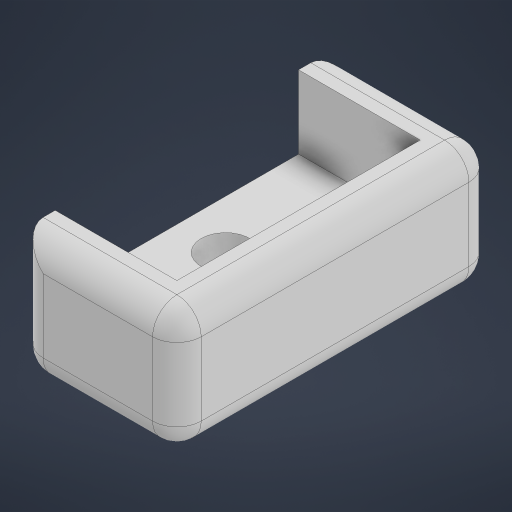
# Autodesk Inventor part: 2
Saved by Autodesk Inventor 2024 (Build 280153000, 153)
## iProperties
Created: 2023-05-05
Part Number: 2
Material: Типовые
Document SubType Name: Modeling
Designer: user
Density: 1 g/cm^3
Appearance: По умолчанию
Author: user
Autodesk Inventor part; units mm, degrees
ref_plane "YZ Plane" through (0, 0, 0) normal (1, 0, 0) x (0, 1, 0)
ref_plane "XZ Plane" through (0, 0, 0) normal (0, 1, 0) x (-1, 0, 0)
ref_plane "XY Plane" through (0, 0, 0) normal (0, 0, 1) x (1, 0, 0)
sketch "Эскиз1" plane through (0, 0, 0) normal (0, 0, 1) x (1, 0, 0)
  line L0 (0, 0) -> (10, 0)
  line L1 (10, 0) -> (10, 20)
  line L2 (10, 20) -> (0, 20)
  line L3 (0, 20) -> (0, 0)
  circle A0 centre (4, 10) radius 2
  point P0 (10, 10)
  dimension "d0" = 10
  dimension "d1" = 4
  dimension "d2" = 6
  dimension "d3" = 20
  constraints: 8 end point, 2 parallel, 1 centre point, 1 horizontal, 1 horizontal alignment, 1 midpoint, 1 perpendicular
  measures "d0" distance of L1.end L2.end
  measures "d1" diameter of A0
  measures "d2" horizontal distance of L1.end A0.centre
  measures "d3" distance of L0.end L1.end
extrude "Выдавливание1" add sketch "Эскиз1" along normal blind 4
sketch "Эскиз2" plane through (0, 0, 4) normal (0, 0, 1) x (1, 0, 0)
  point P0 (0, 0)
sketch "Эскиз3" plane through (0, 0, 0) normal (0, 0, 1) x (1, 0, 0)
  line L0 (0, 23) -> (13, 23)
  line L1 (13, 23) -> (13, -3)
  line L2 (13, -3) -> (0, -3)
  line L3 (0, -3) -> (0, 23)
  line L4 (10, 0) -> (10, 20) projected
  line L5 (10, 20) -> (0, 20) projected
  line L6 (0, 0) -> (10, 0) projected
  point P0 (10, 10)
  point P1 (13, 10)
  dimension "d8" = 3
  dimension "d10" = 3
  constraints: 8 end point, 2 midpoint, 2 parallel, 1 horizontal, 1 horizontal alignment, 1 perpendicular, 1 vertical alignment
  measures "d8" distance from line of L0.end L4
  measures "d10" horizontal distance of L0.end L4.end
extrude "Выдавливание2" add sketch "Эскиз3" along normal blind 10 contours L0 L1 L2 L3 L6 L4 L5
fillet "Сопряжение1" radius 2 11 edges at (13, 10, 0) (6.5, -3, 0) (6.5, 23, 0) (0, 10, 0) (13, 23, 5) (13, 10, 10) (13, -3, 5) (6.5, -3, 10) (6.5, 23, 10) (0, 23, 5) (0, -3, 5)
